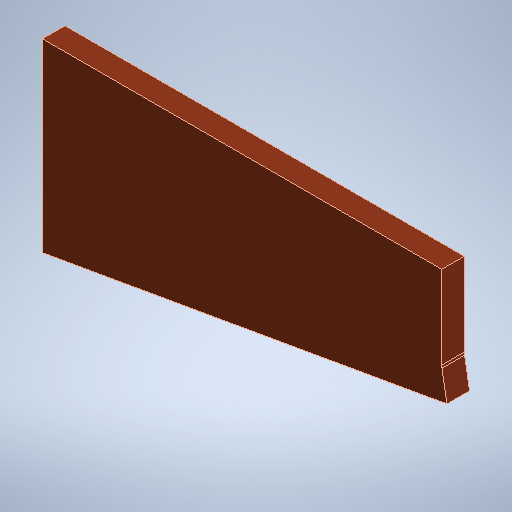
# Autodesk Inventor part: Ramp Side Wall
Saved by Autodesk Inventor 2025.4 (Build 294407000, 407)
## iProperties
Created: 2026-04-06
Part Number: Ramp Side Wall
Material: Generic
Document SubType Name: Sheet Metal
Designer: lenovo
Density: 1 g/cm^3
Sheet Metal Rule: Default_mm
Appearance: Default(1)
Author: lenovo
Autodesk Inventor part; units mm, degrees
ref_plane "YZ Plane" through (0, 0, 0) normal (1, 0, 0) x (0, 1, 0)
ref_plane "XZ Plane" through (0, 0, 0) normal (0, 1, 0) x (-1, 0, 0)
ref_plane "XY Plane" through (0, 0, 0) normal (0, 0, 1) x (1, 0, 0)
sketch "Sketch1" plane through (0, 0, 0) normal (0, 0, 1) x (1, 0, 0)
  line L0 (0, 20) -> (0, 0)
  line L1 (0, 0) -> (50, 8.8163)
  line L2 (0, 20) -> (-3, 20)
  line L3 (-3, 20) -> (-3, -4.5907)
  line L4 (-3, -4.5907) -> (50.6946, 4.8771)
  line L5 (0, 0) -> (50.6946, 0) construction
  line L6 (50, 8.8163) -> (50.6946, 4.8771)
  line L7 (0, 20) -> (50, 20)
  line L8 (50, 20) -> (50, 8.8163)
  line L9 (50.3473, 6.8467) -> (11.5175, 0) construction
  dimension "d0" = 20
  dimension "d1" = 3
  dimension "d2" = 10
  dimension "d3" = 4
  dimension "d4" = 50
  measures "d0" distance of L0.start L0.end
  measures "d1" distance of L0.start L2.end
  measures "d2" angle of L1 L5
  measures "d3" distance of L1.end L4.end
  measures "d4" distance from line of L1.end L0
extrude "Plate1" add sketch "Sketch1" along normal mid plane 3
fillet "Corner Round1" radius 2 1 edges at (50, 8.8163, 0)
equation "\"d5\" = Thickness"
equation "\"BendRadius\" = Thickness"
equation "\"BendReliefWidth\" = Thickness"
equation "\"BendReliefDepth\" = 0.5 * Thickness"
equation "\"CornerReliefSize\" = 4 * Thickness"
equation "\"MinimumRemnant\" = 2 * Thickness"
equation "\"TransitionRadius\" = BendRadius"
equation "\"JacobiRadiusSize\" = BendRadius"
equation "\"GapSize\" = Thickness"
equation "\"Thickness\" = 3"
body "Solid1"
